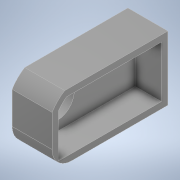
# Autodesk Inventor part: Tilt_Lid
Saved by Autodesk Inventor 2022 (Build 260153000, 153)
## iProperties
Created: 2021-03-07
Part Number: Tilt_Lid
Material: Generic
Document SubType Name: Modeling
Designer: Mlees
Density: 1 g/cm^3
Appearance: Default
Sending System: SolidWorks 2018
Last Author: DELL
Last Saved: 2021-03-08
Nomenclature: 96_Teeth_Gear
Part Number: 96_Teeth_Gear
Source: NOT_KNOWN
Definition: UNKNOWN
Author: Mlees
Revision Number: ANY
Autodesk Inventor part; units mm, degrees
ref_plane "YZ Plane" through (0, 0, 0) normal (1, 0, 0) x (0, 1, 0)
ref_plane "XZ Plane" through (0, 0, 0) normal (0, 1, 0) x (-1, 0, 0)
ref_plane "Work Plane1" through (-5, 30, -18.0278) normal (1, 0, 0) x (0, 0, 1)
sketch "Sketch2" plane through (-5, 30, -18.0278) normal (1, 0, 0) x (0, 0, 1)
  arc A0 (36.0555, 0) -> (48.0278, 11.9722) centre (18.0278, 30) ccw projected
  line L0 (48.0278, 11.9722) -> (48.0278, 48.0278) projected
  arc A1 (36.0555, 0) -> (48.0278, 11.9722) centre (18.0278, 30) ccw
  line L1 (48.0278, 48.0278) -> (48.0278, 11.9722)
  arc A2 (48.0278, 48.0278) -> (36.0555, 60) centre (18.0278, 30) ccw projected
  line L2 (48.0278, 48.0278) -> (48.0278, 60)
  line L3 (48.0278, 60) -> (-61.9722, 60)
  line L4 (-61.9722, 60) -> (-61.9722, 0)
  line L5 (0, 0) -> (36.0555, 0) projected
  line L6 (-61.9722, 0) -> (0, 0)
  line L7 (0, 0) -> (36.0555, 0)
  constraints: 12 end point, 3 perpendicular, 2 point on circle, 2 vertical, 1 centre point, 1 collinear
extrude "Extrusion1" add sketch "Sketch2" along normal blind 26 and the other way blind 2
sketch "Sketch4" plane through (-7, -30, -80) normal (0, -1, 0) x (1, 0, 0)
  line L0 (28, 110) -> (28, 0) projected
  line L1 (0, 0) -> (0, 110) projected
  line L2 (28, 110) -> (0, 110)
  line L3 (0, 110) -> (0, 0)
  line L4 (0, 0) -> (28, 0)
  line L5 (28, 0) -> (28, 110)
  point P0 (7, 80)
  constraints: 8 end point, 2 parallel, 1 horizontal, 1 perpendicular
extrude "Extrusion3" add sketch "Sketch4" along normal blind 1.028
sketch "Sketch5" plane through (21, 30, -18.0278) normal (1, 0, 0) x (0, 0, -1)
  arc A0 (-36.0555, 0) -> (-48.0278, -11.9722) centre (-18.0278, -30) ccw projected
  line L0 (-48.0278, -11.9722) -> (-48.0278, -61.028) projected
  line L1 (-48.0278, -11.9722) -> (-48.0278, -61.028)
  line L2 (61.9722, 0) -> (61.9722, -61.028) projected
  line L3 (-48.0278, -61.028) -> (61.9722, -61.028)
  line L4 (61.9722, -61.028) -> (61.9722, 0)
  line L5 (-36.0555, 0) -> (61.9722, 0) projected
  line L6 (61.9722, 0) -> (-36.0555, 0)
  arc A1 (-36.0555, 0) -> (-48.0278, -11.9722) centre (-18.0278, -30) ccw
  line L7 (55.9722, -55.028) -> (-42.0278, -55.028)
  line L8 (-42.0278, -55.028) -> (-42.0278, -13.7212)
  arc A2 (-34.3066, -6) -> (-42.0278, -13.7212) centre (-18.0278, -30) ccw
  line L9 (-34.3066, -6) -> (55.9722, -6)
  line L10 (55.9722, -6) -> (55.9722, -55.028)
  dimension "d11" = 6
  constraints: 16 end point, 4 perpendicular, 4 point on circle, 2 centre point, 2 collinear, 4 other
  measures "d11" distance between parallel lines of L3 L7
extrude "Extrusion4" cut sketch "Sketch5" against normal blind 25 contours L7 L8 A2 L9 L10
sketch "Sketch6" plane through (-7, 30, -80) normal (-1, 0, 0) x (0, 0, 1)
  line L0 (0, 0) -> (98.0278, 0) projected
  line L1 (0, 0) -> (98.0278, 0)
  line L2 (0, -61.028) -> (110, -61.028) projected
  line L3 (110, -11.9722) -> (110, -61.028)
  line L4 (110, -61.028) -> (0, -61.028)
  line L5 (0, 0) -> (0, -61.028) projected
  line L6 (0, -61.028) -> (0, 0)
  line L7 (110, -11.9722) -> (110, -61.028) projected
  arc A0 (110, -11.9722) -> (98.0278, 0) centre (80, -30) ccw
  point P0 (80, -30)
  constraints: 8 end point, 2 collinear, 2 point on circle, 1 centre point, 1 horizontal, 1 perpendicular
extrude "Extrusion5" add sketch "Sketch6" along normal blind 10
sketch "Sketch7" plane through (-17, 30, -80) normal (-1, 0, 0) x (0, 0, 1)
  circle A0 centre (80, -30) radius 16.05
  dimension "d16" = 32.1
  constraints: 1 centre point, 1 coincident
  measures "d16" diameter of A0
extrude "Extrusion6" cut sketch "Sketch7" against normal blind 13
fillet "Fillet1" radius 18.5 1 edges at (2, -31.028, 30)
body "Solid1"
